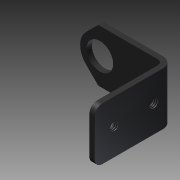
# Autodesk Inventor part: D-025
Saved by Autodesk Inventor 2015 (Build 190159000, 159)
## iProperties
Company: MARCHA TECHNOLOGY
Created: 2013-09-28
Part Number: D-025
Document SubType Name: Chapa
Designer: O.Martin
Density: 7.85 g/cm^3
Project: WITBOXprinter_K01
Stock Number: 28655
Material: Steel
Description: SOPORTE RODAMIENTO Z
Mass: 23.2596 g
Surface Area: 33.7201 cm^2
Volume: 2.963 cm^3
Sheet Metal Rule: Por defecto
Appearance: Rubber - Black - Version 1.1
Author: O.Martin
Autodesk Inventor part; units mm, degrees
ref_plane "YZ Plane" through (0, 0, 0) normal (1, 0, 0) x (0, 1, 0)
ref_plane "XZ Plane" through (0, 0, 0) normal (0, 1, 0) x (-1, 0, 0)
ref_plane "XY Plane" through (0, 0, 0) normal (0, 0, 1) x (1, 0, 0)
sketch "Boceto1" plane through (0, 0, 0) normal (0, 0, 1) x (1, 0, 0)
  line L0 (3.6818, 62.9397) -> (3.6818, 22.9397)
  line L1 (3.6818, 22.9397) -> (-43.3182, 22.9397)
  line L2 (-43.3182, 22.9397) -> (-43.3182, 24.9397)
  line L3 (-43.3182, 24.9397) -> (1.6818, 24.9397)
  line L4 (1.6818, 24.9397) -> (1.6818, 60.9397)
  line L5 (1.6818, 60.9397) -> (-29.8182, 60.9397)
  line L6 (-29.8182, 60.9397) -> (-29.8182, 62.9397)
  line L7 (-29.8182, 62.9397) -> (3.6818, 62.9397)
  dimension "d2" = 2
  dimension "d3" = 47
  dimension "d6" = 2
  dimension "d40" = 2
  dimension "d42" = 40
  dimension "d60" = 13.5
  constraints: 16 end point, 4 parallel, 3 perpendicular, 1 vertical
  measures "d2" distance between parallel lines of L0 L4
  measures "d3" distance of L0.end L1.end
  measures "d6" distance of L1.end L2.end
  measures "d40" distance of L5.end L6.end
  measures "d42" distance of L0.start L0.end
  measures "d60" distance between parallel lines of L2 L6
extrude "Extrusión1" add sketch "Boceto1" along normal mid plane 42.5
sketch "Boceto2" plane through (3.6818, 22.9397, 21.25) normal (1, 0, 0) x (0, 0, -1)
  line L0 (0, 0) -> (42.5, 0) projected
  line L1 (8.75, 7.5) -> (33.75, 7.5) construction
  line L2 (33.75, 7.5) -> (33.75, 32.5) construction
  line L3 (33.75, 32.5) -> (8.75, 32.5) construction
  line L4 (8.75, 32.5) -> (8.75, 7.5) construction
  line L5 (42.5, 40) -> (0, 40) projected
  point P0 (21.25, 7.5)
  point P1 (21.25, 0)
  point P2 (8.75, 20)
  point P3 (21.25, 17.5)
  point P4 (21.25, 32.5)
  point P5 (21.25, 32.5)
  dimension "d54" = 25
  dimension "d55" = 25
  dimension "d70" = 15
  dimension "d76" = 7.5
  constraints: 8 end point, 4 coincident, 4 midpoint, 2 parallel, 2 vertical alignment, 1 horizontal, 1 perpendicular
  measures "d54" distance of L1.start L1.end
  measures "d55" distance of L3.end L1.start
  measures "d70" distance from line of L3 point (21.25, 17.5)
  measures "d76" distance between parallel lines of L5 L3
hole "Agujero1" at (3.6818, 40.4397, 0) at (3.6818, 55.4397, 0) direction (-1, 0, 0) diameter 3.242 end through all thread size "M4x0.7" class "6H" standard "ISO Metric profile"
sketch "Boceto3" plane through (-43.3182, 22.9397, 21.25) normal (0, -1, 0) x (1, 0, 0)
  line L0 (0, -42.5) -> (0, 0) projected
  line L1 (47, 0) -> (47, -42.5) projected
  circle A0 centre (23.5, -21.25) radius 11.05
  line L2 (39, -36.75) -> (8, -36.75) construction
  line L3 (8, -36.75) -> (8, -5.75) construction
  line L4 (8, -5.75) -> (39, -5.75) construction
  line L5 (39, -5.75) -> (39, -36.75) construction
  point P0 (0, -21.25)
  point P1 (8, -21.25)
  point P2 (23.5, -36.75)
  dimension "d17" = 23.5
  dimension "d18" = 22.1
  dimension "d19" = 31
  constraints: 8 end point, 4 coincident, 3 midpoint, 2 horizontal alignment, 2 parallel, 2 perpendicular, 1 centre point, 1 horizontal, 1 vertical alignment
  measures "d17" distance from line of L1 A0.centre
  measures "d18" diameter of A0
  measures "d19" distance of L2.end L3.end
hole "Agujero2" at (-4.3182, 22.9397, -15.5) at (-35.3182, 22.9397, -15.5) at (-35.3182, 22.9397, 15.5) at (-4.3182, 22.9397, 15.5) direction (0, 1, 0) diameter 3.5 depth 8 tip angle 118
extrude "Extrusión2" cut sketch "Boceto3" against normal blind 2
fillet "Empalme1" radius 4 2 edges at (3.6818, 22.9397, 0) (3.6818, 62.9397, 0)
fillet "Empalme1" radius 2 2 edges at (1.6818, 24.9397, 0) (1.6818, 60.9397, 0)
chamfer "Chaflán1" distance 4 angle 45 4 edges at (-43.3182, 23.9397, -21.25) (-43.3182, 23.9397, 21.25) (-29.8182, 61.9397, -21.25) (-29.8182, 61.9397, 21.25)
ref_plane "Plano de trabajo1" through (-44.2845, 22.9397, -21.15) normal (0, 1, 0) x (0, 0, 1)
sketch "Boceto6" plane through (-0.3182, 62.9397, 21.25) normal (0, 1, 0) x (1, 0, 0)
  line L0 (-29.5, 38.5) -> (-29.5, 4) projected
  line L1 (4, 0) -> (4, 42.5) projected
  point P0 (-22, 21.25)
  point P1 (-29.5, 21.25)
  dimension "d61" = 7.5
  constraints: 1 horizontal alignment, 1 midpoint
  measures "d61" distance from line of L0 point (-22, 21.25)
hole "Agujero3" at (-22.3182, 62.9397, 0) direction (0, -1, 0) diameter 10.1 depth 8 tip angle 118
sketch "Boceto7" plane through (-0.3182, 62.9397, 21.25) normal (0, 1, 0) x (1, 0, 0)
  circle A0 centre (-22, 21.25) radius 5.05 projected
  line L0 (-29.5, 38.5) -> (-25.5, 42.5) projected
  line L1 (-29.5, 38.5) -> (-29.5, 4) projected
  line L2 (-25.5, 0) -> (-29.5, 4) projected
  line L3 (-25.5, 0) -> (0, 0) projected
  line L4 (0, 42.5) -> (-25.5, 42.5) projected
  circle A1 centre (-22, 21.25) radius 7.5
  line L5 (-27.3033, 15.9467) -> (-11.3566, 0)
  line L6 (-27.3033, 26.5533) -> (-11.3566, 42.5)
  constraints: 4 end point, 3 tangent, 2 parallel, 2 point on circle, 2 point on line, 1 centre point, 1 coincident
extrude "Extrusión5" cut sketch "Boceto7" against normal blind 10 contours L0 L4 L6 A1 L1 | A1 L5 L3 L2 L1
fillet "Empalme2" radius 4 2 edges at (-11.6749, 61.9397, -21.25) (-11.6749, 61.9397, 21.25)
sketch "Boceto8" plane through (3.6818, 26.9397, 21.25) normal (1, 0, 0) x (0, 0, -1)
  line L0 (-20.0023, 6) -> (90.3575, 6)
  line L1 (90.3575, 6) -> (90.3575, -39.4448)
  line L2 (90.3575, -39.4448) -> (-20.0023, -39.4448)
  line L3 (-20.0023, -39.4448) -> (-20.0023, 6)
  line L4 (42.5, 36) -> (0, 36) projected
  dimension "d56" = 30
  constraints: 8 end point, 2 parallel, 1 horizontal, 1 perpendicular
  measures "d56" distance between parallel lines of L4 L0
extrude "Extrusión6" cut sketch "Boceto8" against normal through all
sketch "Boceto9" plane through (-0.3182, 62.9397, 21.25) normal (0, 1, 0) x (1, 0, 0)
  line L0 (0, 42.5) -> (-9.6997, 42.5) projected
  arc A0 (-27.3033, 26.5533) -> (-27.3033, 15.9467) centre (-22, 21.25) ccw projected
  circle A1 centre (-22, 21.25) radius 5.05 projected
  circle A2 centre (-22, 21.25) radius 5.25
  line L1 (-22, 16.2) -> (-22, 26.3) construction
  line L2 (-26.3734, 18.725) -> (-17.6266, 23.775) construction
  line L3 (-26.3734, 23.775) -> (-17.6266, 18.725) construction
  line L4 (-26.3734, 18.725) -> (-26.5466, 18.625)
  line L5 (-26.3734, 23.775) -> (-26.5466, 23.875)
  line L6 (-17.6266, 23.775) -> (-17.4534, 23.875)
  line L7 (-22, 26.3) -> (-22, 26.5)
  line L8 (-17.6266, 18.725) -> (-17.4534, 18.625)
  line L9 (-22, 16.2) -> (-22, 16)
  dimension "d62" = 60
  dimension "d63" = 60
  dimension "d64" = 0.2
  constraints: 18 end point, 12 point on circle, 6 collinear, 3 coincident, 3 midpoint, 1 centre point, 1 perpendicular
  measures "d62" angle of L1 L2
  measures "d63" angle of L1 L3
  measures "d64" radial gap between concentric circles of A1 A2
extrude "Extrusión7" [suppressed]
fillet "Empalme3" radius 4 2 edges at (2.6818, 32.9397, -21.25) (2.6818, 32.9397, 21.25)
sketch "Boceto10" plane through (1.6818, 58.9397, -21.25) normal (-1, 0, 0) x (0, 0, 1)
  line L0 (4, -26) -> (38.5, -26) projected
  circle A0 centre (8.75, -3.5) radius 1.621 projected
  line L1 (7.75, -26) -> (8.75, -25)
  line L2 (8.75, -25) -> (9.75, -26)
  dimension "d67" = 1
  constraints: 4 end point, 2 perpendicular, 2 point on line, 1 vertical alignment
  measures "d67" distance from line of L0 L1.end
extrude "Extrusión8" cut sketch "Boceto10" against normal through all contours L1 L2 L0
sketch "Boceto12" plane through (-0.3182, 62.9397, 21.25) normal (0, 1, 0) x (1, 0, 0)
  arc A0 (-27.3033, 26.5533) -> (-27.3033, 15.9467) centre (-22, 21.25) ccw projected
  circle A1 centre (-22, 21.25) radius 5.05 projected
  line L0 (15.817, 31.25) -> (-45.8326, 31.25)
  line L1 (-45.8326, 31.25) -> (-45.8326, 11.25)
  line L2 (-45.8326, 11.25) -> (15.817, 11.25)
  line L3 (15.817, 11.25) -> (15.817, 31.25)
  point P0 (-45.8326, 21.25)
  dimension "d77" = 20
  constraints: 8 end point, 2 parallel, 1 horizontal, 1 horizontal alignment, 1 midpoint, 1 perpendicular
  measures "d77" distance of L2.end L0.start
extrude "Extrusión10" cut sketch "Boceto12" against normal through all contours A1 | L3 L2 L1 L0 keep common part
fillet "Redondeo de esquina1" radius 3 2 edges at (2.6818, 32.9397, -10) (2.6818, 32.9397, 10)
equation "\"d2\" = d1"
equation "\"d63\" = d62"
equation "\"Radio_pliegue\" = Grosor"
equation "\"Anchura_desahogo_plegado\" = Grosor"
equation "\"Profundidad_desahogo_plegado\" = 0.5 * Grosor"
equation "\"Tamaño_destalonado\" = 4 * Grosor"
equation "\"Remanente_mínimo\" = 2 * Grosor"
equation "\"Radiodetransición\" = Radio_pliegue"
equation "\"Tamaño_de_radio_de_Jacobi\" = Grosor"
equation "\"GapSize\" = Grosor"
equation "\"d1\" = 2"
equation "\"Grosor\" = 2"
body "Solid1"
